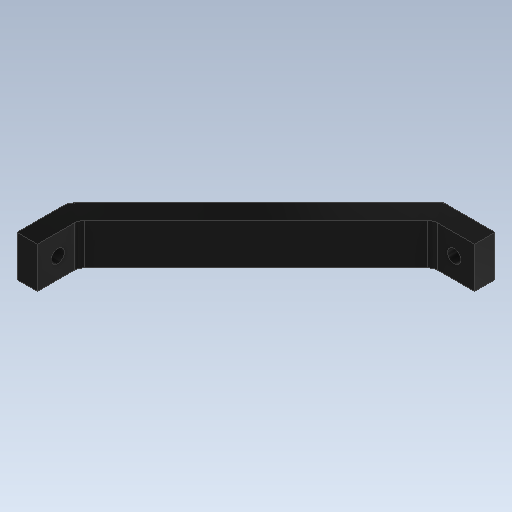
# Autodesk Inventor part: 0008-10-025 Ranforsare 2
Saved by Autodesk Inventor 2020 (Build 240168000, 168)
## iProperties
Created: 2020-12-09
Part Number: 0008-10-025 Ranforsare 2
Material: ABS Plastic
Document SubType Name: Modeling
Designer: Botoca
Mass: 37.2847 g
Surface Area: 111.051 cm^2
Volume: 35.1743 cm^3
Density: 1.06 g/cm^3
Appearance: Smooth - White
Author: Botoca
Autodesk Inventor part; units mm, degrees
ref_plane "YZ Plane" through (0, 0, 0) normal (1, 0, 0) x (0, 1, 0)
ref_plane "XZ Plane" through (0, 0, 0) normal (0, 1, 0) x (-1, 0, 0)
ref_plane "XY Plane" through (0, 0, 0) normal (0, 0, 1) x (1, 0, 0)
sketch "Sketch1" plane through (0, 0, 0) normal (0, 0, 1) x (1, 0, 0)
  line L0 (0, 0) -> (0, 25)
  line L1 (0, 25) -> (91.9239, 116.9239)
  line L2 (91.9239, 116.9239) -> (116.9239, 116.9239)
  line L3 (-11.5144, -3.3847) -> (12.7866, -3.3847) construction
  line L4 (116.9239, 116.9239) -> (116.9239, 106.9239)
  line L5 (116.9239, 106.9239) -> (96.9239, 106.9239)
  line L6 (96.9239, 106.9239) -> (10, 20)
  line L7 (10, 20) -> (10, 0)
  line L8 (10, 0) -> (0, 0)
  dimension "d0" = 90
  dimension "d1" = 25
  dimension "d4" = 45
  dimension "d5" = 130
  dimension "d6" = 10
  dimension "d7" = 10
  dimension "d26" = 96.9239
  dimension "d27" = 25
  constraints: 18 end point, 4 perpendicular, 2 coincident, 2 horizontal, 1 parallel, 1 point on line
  measures "d0" angle of L2 L0
  measures "d1" distance of L0.start L0.end
  measures "d4" angle of L0 L1
  measures "d5" distance of L1.end L0.end
  measures "d6" distance of L2.end L4.end
  measures "d7" distance of L7.end L0.start
  measures "d26" horizontal distance of point (0, 0) L5.end
  measures "d27" distance of L1.end L2.end
extrude "Extrusion1" add sketch "Sketch1" along normal blind 20
sketch "Sketch2" plane through (10, 0, 0) normal (1, 0, 0) x (0, 0, -1)
  line L0 (0, 0) -> (-20, 0) projected
  line L1 (-20, 0) -> (-20, 20) projected
  point P0 (-10, 10)
  point P1 (-10, 0)
  point P2 (-20, 10)
  constraints: 2 midpoint, 1 horizontal alignment, 1 vertical alignment
sketch "Sketch3" plane through (96.9239, 106.9239, 0) normal (0, -1, 0) x (1, 0, 0)
  line L0 (0, 20) -> (20, 20) projected
  line L1 (20, 0) -> (20, 20) projected
  point P0 (-96.9239, 0)
  point P1 (10, 10)
  point P2 (10, 20)
  point P3 (20, 10)
  constraints: 2 midpoint, 1 horizontal alignment, 1 vertical alignment
hole "Hole1" at (10, 10, 10) direction (-1, 0, 0) diameter 6.5 end through all
hole "Hole2" at (106.9239, 106.9239, 10) direction (0, 1, 0) diameter 6.5 end through all
fillet "Fillet1" radius 5 3 edges at (10, 20, 10) (0, 25, 10) (96.9239, 106.9239, 10)
body "Solid1"
